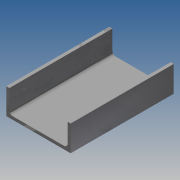
# Autodesk Inventor part: 2p0ch37
Saved by Autodesk Inventor 2013 (Build 170138000, 138)
## iProperties
Company: HERA Project
Created: 2013-12-03
Part Number: 2p0ch37
Material: Steel, Galvanized
Document SubType Name: Modeling
Designer: David DeBoer
Mass: 266.491 g
Surface Area: 229.978 cm^2
Volume: 33.9479 cm^3
Density: 7.85 g/cm^3
Description: metal end channel 37 degrees
Author: David DeBoer
Autodesk Inventor part; units mm, degrees
ref_plane "YZ Plane" through (0, 0, 0) normal (1, 0, 0) x (0, 1, 0)
ref_plane "XZ Plane" through (0, 0, 0) normal (0, 1, 0) x (-1, 0, 0)
ref_plane "XY Plane" through (0, 0, 0) normal (0, 0, 1) x (1, 0, 0)
sketch "Sketch1" plane through (0, 0, 0) normal (0, 0, 1) x (1, 0, 0)
  line L0 (0, 0) -> (63.5, 0)
  line L1 (0, 0) -> (0, 25.4)
  line L2 (63.5, 0) -> (63.5, 25.4)
  line L3 (60.452, 25.4) -> (60.452, 6.223)
  line L4 (57.277, 3.048) -> (6.223, 3.048)
  line L5 (3.048, 6.223) -> (3.048, 25.4)
  line L6 (0, 25.4) -> (3.048, 25.4)
  line L7 (60.452, 25.4) -> (63.5, 25.4)
  arc A0 (3.048, 6.223) -> (6.223, 3.048) centre (6.223, 6.223) ccw
  arc A1 (57.277, 3.048) -> (60.452, 6.223) centre (57.277, 6.223) ccw
  dimension "d0" = 63.5
  dimension "d1" = 25.4
  dimension "d2" = 3.048
  dimension "d3" = 3.175
  constraints: 16 end point, 4 point on circle, 4 tangent, 3 equal length, 3 perpendicular, 2 centre point, 1 equal radius, 2 other
  measures "d0" distance of L0.start L0.end
  measures "d1" distance of L0.start L1.end
  measures "d2" distance between parallel lines of L0 L4
  measures "d3" radius of A0
extrude "Extrusion1" add sketch "Sketch1" along normal blind 101.6
body "Solid1"
